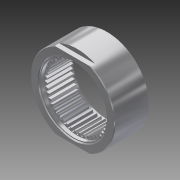
# Autodesk Inventor part: P60 Ring Gear 1-Stage
Saved by Autodesk Inventor 2014 SP1 (Build 180222100, 222)
## iProperties
Created: 2012-01-14
Part Number: P60 Ring Gear 1-Stage
Material: Aluminum 6061
Document SubType Name: Modeling
Designer: Moses
Density: 2.71 g/cm^3
Mass: 18.5911 g
Surface Area: 48.1148 cm^2
Volume: 6.86017 cm^3
Appearance: Aluminum - Polished
Author: Moses
Autodesk Inventor part; units mm, degrees
ref_plane "YZ Plane" through (0, 0, 0) normal (1, 0, 0) x (0, 1, 0)
ref_plane "XZ Plane" through (0, 0, 0) normal (0, 1, 0) x (-1, 0, 0)
sketch "Sketch1" plane through (0, 0, 0) normal (0, 0, 1) x (1, 0, 0)
  circle A0 centre (0, 0) radius 18.415
  circle A1 centre (0, 0) radius 14.9225
  dimension "d0" = 36.83
  dimension "d1" = 29.845
  constraints: 2 centre point, 2 coincident
  measures "d0" diameter of A0
  measures "d1" diameter of A1
extrude "Extrusion1" add sketch "Sketch1" along normal blind 15.24
chamfer "Chamfer1" distance 0.254 angle 45 4 edges at (-18.415, 0, 15.24) (-14.9225, 0, 15.24) (-18.415, 0, 0) (-14.9225, 0, 0)
sketch "Sketch2" plane through (0, 0, 15.24) normal (0, 0, 1) x (1, 0, 0)
  circle A0 centre (0, 0) radius 18.415 projected
  line L0 (-7.9375, 16.6165) -> (7.9375, 16.6165)
  line L1 (-7.9375, -16.6165) -> (7.9375, -16.6165)
  dimension "d7" = 15.875
  dimension "d16" = 36.83
  constraints: 4 end point, 4 point on circle, 2 parallel, 1 horizontal
  measures "d7" distance of L1.start L1.end
  measures "d16" diameter of A0
extrude "Extrusion2" cut sketch "Sketch2" against normal blind 2 contours L0 A0 | A0 L1
ref_plane "Work Plane1" through (0, 0, 7.62) normal (0, 0, 1) x (1, 0, 0)
sketch "Sketch3" plane through (0, 0, 7.62) normal (0, 0, 1) x (1, 0, 0)
  arc A0 (2.2292, -14.0746) -> (2.4908, -12.8141) centre (-3.3575, -12.2576) ccw
  arc A1 (1.7366, -14.1438) -> (2.2292, -14.0746) centre (0, 0) ccw
  arc A2 (1.1377, -13.0043) -> (1.7366, -14.1438) centre (6.6061, -10.8573) ccw
  arc A3 (0.6832, -13.0361) -> (1.1377, -13.0043) centre (0, 0) ccw
  arc A4 (0.2487, -14.2478) -> (0.6832, -13.0361) centre (-5.0308, -11.671) ccw
  arc A5 (-0.2487, -14.2478) -> (0.2487, -14.2478) centre (0, 0) ccw
  arc A6 (-0.6832, -13.0361) -> (-0.2487, -14.2478) centre (5.0308, -11.671) ccw
  arc A7 (-1.1377, -13.0043) -> (-0.6832, -13.0361) centre (0, 0) ccw
  arc A8 (-1.7366, -14.1438) -> (-1.1377, -13.0043) centre (-6.6061, -10.8573) ccw
  arc A9 (-2.2292, -14.0746) -> (-1.7366, -14.1438) centre (0, 0) ccw
  arc A10 (-2.4908, -12.8141) -> (-2.2292, -14.0746) centre (3.3575, -12.2576) ccw
  arc A11 (-2.9365, -12.7194) -> (-2.4908, -12.8141) centre (0, 0) ccw
  arc A12 (-3.6882, -13.7644) -> (-2.9365, -12.7194) centre (-8.0529, -9.8322) ccw
  arc A13 (-4.1663, -13.6273) -> (-3.6882, -13.7644) centre (0, 0) ccw
  arc A14 (-4.25, -12.3428) -> (-4.1663, -13.6273) centre (1.6189, -12.6056) ccw
  arc A15 (-4.6781, -12.1869) -> (-4.25, -12.3428) centre (0, 0) ccw
  arc A16 (-5.5679, -13.1172) -> (-4.6781, -12.1869) centre (-9.3429, -8.6158) ccw
  arc A17 (-6.0223, -12.9149) -> (-5.5679, -13.1172) centre (0, 0) ccw
  arc A18 (-5.9264, -11.6312) -> (-6.0223, -12.9149) centre (-0.1512, -12.7082) ccw
  arc A19 (-6.3287, -11.4173) -> (-5.9264, -11.6312) centre (0, 0) ccw
  arc A20 (-7.3393, -12.2146) -> (-6.3287, -11.4173) centre (-10.451, -7.2317) ccw
  arc A21 (-7.7611, -11.9511) -> (-7.3393, -12.2146) centre (0, 0) ccw
  arc A22 (-7.4874, -10.6932) -> (-7.7611, -11.9511) centre (-1.9183, -12.5635) ccw
  arc A23 (-7.8561, -10.4254) -> (-7.4874, -10.6932) centre (0, 0) ccw
  arc A24 (-8.9678, -11.0743) -> (-7.8561, -10.4254) centre (-11.3558, -5.7068) ccw
  arc A25 (-9.3488, -10.7546) -> (-8.9678, -11.0743) centre (0, 0) ccw
  arc A26 (-8.9028, -9.5471) -> (-9.3488, -10.7546) centre (-3.6482, -12.1742) ccw
  arc A27 (-9.2305, -9.2305) -> (-8.9028, -9.5471) centre (0, 0) ccw
  arc A28 (-10.4218, -9.7185) -> (-9.2305, -9.2305) centre (-12.0395, -4.0708) ccw
  arc A29 (-10.7546, -9.3488) -> (-10.4218, -9.7185) centre (0, 0) ccw
  arc A30 (-10.1448, -8.2151) -> (-10.7546, -9.3488) centre (-5.307, -11.548) ccw
  arc A31 (-10.4254, -7.8561) -> (-10.1448, -8.2151) centre (0, 0) ccw
  arc A32 (-11.6729, -8.1735) -> (-10.4254, -7.8561) centre (-12.4889, -2.3556) ccw
  arc A33 (-11.9511, -7.7611) -> (-11.6729, -8.1735) centre (0, 0) ccw
  arc A34 (-11.1894, -6.7233) -> (-11.9511, -7.7611) centre (-6.8625, -10.6971) ccw
  arc A35 (-11.4173, -6.3287) -> (-11.1894, -6.7233) centre (0, 0) ccw
  arc A36 (-12.6968, -6.4694) -> (-11.4173, -6.3287) centre (-12.6952, -0.5946) ccw
  arc A37 (-12.9149, -6.0223) -> (-12.6968, -6.4694) centre (0, 0) ccw
  arc A38 (-12.0162, -5.1006) -> (-12.9149, -6.0223) centre (-8.2845, -9.6379) ccw
  arc A39 (-12.1869, -4.6781) -> (-12.0162, -5.1006) centre (0, 0) ccw
  arc A40 (-13.4736, -4.6393) -> (-12.1869, -4.6781) centre (-12.6544, 1.178) ccw
  arc A41 (-13.6273, -4.1663) -> (-13.4736, -4.6393) centre (0, 0) ccw
  arc A42 (-12.6092, -3.3786) -> (-13.6273, -4.1663) centre (-9.5452, -8.3911) ccw
  arc A43 (-12.7194, -2.9365) -> (-12.6092, -3.3786) centre (0, 0) ccw
  arc A44 (-13.9882, -2.719) -> (-12.7194, -2.9365) centre (-12.3673, 2.9277) ccw
  arc A45 (-14.0746, -2.2292) -> (-13.9882, -2.719) centre (0, 0) ccw
  arc A46 (-12.9567, -1.5909) -> (-14.0746, -2.2292) centre (-10.6201, -6.981) ccw
  arc A47 (-13.0043, -1.1377) -> (-12.9567, -1.5909) centre (0, 0) ccw
  arc A48 (-14.2305, -0.7458) -> (-13.0043, -1.1377) centre (-11.8395, 4.6204) ccw
  arc A49 (-14.2478, -0.2487) -> (-14.2305, -0.7458) centre (0, 0) ccw
  arc A50 (-13.052, 0.2278) -> (-14.2478, -0.2487) centre (-11.4883, -5.435) ccw
  arc A51 (-13.0361, 0.6832) -> (-13.052, 0.2278) centre (0, 0) ccw
  arc A52 (-14.1958, 1.242) -> (-13.0361, 0.6832) centre (-11.0812, 6.2232) ccw
  arc A53 (-14.1438, 1.7366) -> (-14.1958, 1.242) centre (0, 0) ccw
  arc A54 (-12.8932, 2.0421) -> (-14.1438, 1.7366) centre (-12.1329, -3.7833) ccw
  arc A55 (-12.8141, 2.4908) -> (-12.8932, 2.0421) centre (0, 0) ccw
  arc A56 (-13.8848, 3.2056) -> (-12.8141, 2.4908) centre (-10.1073, 7.7048) ccw
  arc A57 (-13.7644, 3.6882) -> (-13.8848, 3.2056) centre (0, 0) ccw
  arc A58 (-12.4836, 3.8166) -> (-13.7644, 3.6882) centre (-12.5414, -2.0579) ccw
  arc A59 (-12.3428, 4.25) -> (-12.4836, 3.8166) centre (0, 0) ccw
  arc A60 (-13.3035, 5.1067) -> (-12.3428, 4.25) centre (-8.9366, 9.0365) ccw
  arc A61 (-13.1172, 5.5679) -> (-13.3035, 5.1067) centre (0, 0) ccw
  arc A62 (-11.8309, 5.5168) -> (-13.1172, 5.5679) centre (-12.7057, -0.2924) ccw
  arc A63 (-11.6312, 5.9264) -> (-11.8309, 5.5168) centre (0, 0) ccw
  arc A64 (-12.4633, 6.9085) -> (-11.6312, 5.9264) centre (-7.592, 10.1923) ccw
  arc A65 (-12.2146, 7.3393) -> (-12.4633, 6.9085) centre (0, 0) ccw
  arc A66 (-10.948, 7.1097) -> (-12.2146, 7.3393) centre (-12.6228, 1.4787) ccw
  arc A67 (-10.6932, 7.4874) -> (-10.948, 7.1097) centre (0, 0) ccw
  arc A68 (-11.3806, 8.5759) -> (-10.6932, 7.4874) centre (-6.0996, 11.1497) ccw
  arc A69 (-11.0743, 8.9678) -> (-11.3806, 8.5759) centre (0, 0) ccw
  arc A70 (-9.852, 8.5642) -> (-11.0743, 8.9678) centre (-12.2941, 3.2211) ccw
  arc A71 (-9.5471, 8.9028) -> (-9.852, 8.5642) centre (0, 0) ccw
  arc A72 (-10.0763, 10.0763) -> (-9.5471, 8.9028) centre (-4.4885, 11.8901) ccw
  arc A73 (-9.7185, 10.4218) -> (-10.0763, 10.0763) centre (0, 0) ccw
  arc A74 (-8.5642, 9.852) -> (-9.7185, 10.4218) centre (-11.7262, 4.9007) ccw
  arc A75 (-8.2151, 10.1448) -> (-8.5642, 9.852) centre (0, 0) ccw
  arc A76 (-8.5759, 11.3806) -> (-8.2151, 10.1448) centre (-2.79, 12.3991) ccw
  arc A77 (-8.1735, 11.6729) -> (-8.5759, 11.3806) centre (0, 0) ccw
  arc A78 (-7.1097, 10.948) -> (-8.1735, 11.6729) centre (-10.93, 6.485) ccw
  arc A79 (-6.7233, 11.1894) -> (-7.1097, 10.948) centre (0, 0) ccw
  arc A80 (-6.9085, 12.4633) -> (-6.7233, 11.1894) centre (-1.0373, 12.6667) ccw
  arc A81 (-6.4694, 12.6968) -> (-6.9085, 12.4633) centre (0, 0) ccw
  arc A82 (-5.5168, 11.8309) -> (-6.4694, 12.6968) centre (-9.9211, 7.9431) ccw
  arc A83 (-5.1006, 12.0162) -> (-5.5168, 11.8309) centre (0, 0) ccw
  arc A84 (-5.1067, 13.3035) -> (-5.1006, 12.0162) centre (0.7357, 12.6878) ccw
  arc A85 (-4.6393, 13.4736) -> (-5.1067, 13.3035) centre (0, 0) ccw
  arc A86 (-3.8166, 12.4836) -> (-4.6393, 13.4736) centre (-8.7191, 9.2465) ccw
  arc A87 (-3.3786, 12.6092) -> (-3.8166, 12.4836) centre (0, 0) ccw
  arc A88 (-3.2056, 13.8848) -> (-3.3786, 12.6092) centre (2.4943, 12.4619) ccw
  arc A89 (-2.719, 13.9882) -> (-3.2056, 13.8848) centre (0, 0) ccw
  arc A90 (-2.0421, 12.8932) -> (-2.719, 13.9882) centre (-7.3474, 10.37) ccw
  arc A91 (-1.5909, 12.9567) -> (-2.0421, 12.8932) centre (0, 0) ccw
  arc A92 (-1.242, 14.1958) -> (-1.5909, 12.9567) centre (4.2044, 11.9935) ccw
  arc A93 (-0.7458, 14.2305) -> (-1.242, 14.1958) centre (0, 0) ccw
  arc A94 (-0.2278, 13.052) -> (-0.7458, 14.2305) centre (-5.8327, 11.2916) ccw
  arc A95 (0.2278, 13.052) -> (-0.2278, 13.052) centre (0, 0) ccw
  arc A96 (0.7458, 14.2305) -> (0.2278, 13.052) centre (5.8327, 11.2916) ccw
  arc A97 (1.242, 14.1958) -> (0.7458, 14.2305) centre (0, 0) ccw
  arc A98 (1.5909, 12.9567) -> (1.242, 14.1958) centre (-4.2044, 11.9935) ccw
  arc A99 (2.0421, 12.8932) -> (1.5909, 12.9567) centre (0, 0) ccw
  arc A100 (2.719, 13.9882) -> (2.0421, 12.8932) centre (7.3474, 10.37) ccw
  arc A101 (3.2056, 13.8848) -> (2.719, 13.9882) centre (0, 0) ccw
  arc A102 (3.3786, 12.6092) -> (3.2056, 13.8848) centre (-2.4943, 12.4619) ccw
  arc A103 (3.8166, 12.4836) -> (3.3786, 12.6092) centre (0, 0) ccw
  arc A104 (4.6393, 13.4736) -> (3.8166, 12.4836) centre (8.7191, 9.2465) ccw
  arc A105 (5.1067, 13.3035) -> (4.6393, 13.4736) centre (0, 0) ccw
  arc A106 (5.1006, 12.0162) -> (5.1067, 13.3035) centre (-0.7357, 12.6878) ccw
  arc A107 (5.5168, 11.8309) -> (5.1006, 12.0162) centre (0, 0) ccw
  arc A108 (6.4694, 12.6968) -> (5.5168, 11.8309) centre (9.9211, 7.9431) ccw
  arc A109 (6.9085, 12.4633) -> (6.4694, 12.6968) centre (0, 0) ccw
  arc A110 (6.7233, 11.1894) -> (6.9085, 12.4633) centre (1.0373, 12.6667) ccw
  arc A111 (7.1097, 10.948) -> (6.7233, 11.1894) centre (0, 0) ccw
  arc A112 (8.1735, 11.6729) -> (7.1097, 10.948) centre (10.93, 6.485) ccw
  arc A113 (8.5759, 11.3806) -> (8.1735, 11.6729) centre (0, 0) ccw
  arc A114 (8.2151, 10.1448) -> (8.5759, 11.3806) centre (2.79, 12.3991) ccw
  arc A115 (8.5642, 9.852) -> (8.2151, 10.1448) centre (0, 0) ccw
  arc A116 (9.7185, 10.4218) -> (8.5642, 9.852) centre (11.7262, 4.9007) ccw
  arc A117 (10.0763, 10.0763) -> (9.7185, 10.4218) centre (0, 0) ccw
  arc A118 (9.5471, 8.9028) -> (10.0763, 10.0763) centre (4.4885, 11.8901) ccw
  arc A119 (9.852, 8.5642) -> (9.5471, 8.9028) centre (0, 0) ccw
  arc A120 (11.0743, 8.9678) -> (9.852, 8.5642) centre (12.2941, 3.2211) ccw
  arc A121 (11.3806, 8.5759) -> (11.0743, 8.9678) centre (0, 0) ccw
  arc A122 (10.6932, 7.4874) -> (11.3806, 8.5759) centre (6.0996, 11.1497) ccw
  arc A123 (10.948, 7.1097) -> (10.6932, 7.4874) centre (0, 0) ccw
  arc A124 (12.2146, 7.3393) -> (10.948, 7.1097) centre (12.6228, 1.4787) ccw
  arc A125 (12.4633, 6.9085) -> (12.2146, 7.3393) centre (0, 0) ccw
  arc A126 (11.6312, 5.9264) -> (12.4633, 6.9085) centre (7.592, 10.1923) ccw
  arc A127 (11.8309, 5.5168) -> (11.6312, 5.9264) centre (0, 0) ccw
  arc A128 (13.1172, 5.5679) -> (11.8309, 5.5168) centre (12.7057, -0.2924) ccw
  arc A129 (13.3035, 5.1067) -> (13.1172, 5.5679) centre (0, 0) ccw
  arc A130 (12.3428, 4.25) -> (13.3035, 5.1067) centre (8.9366, 9.0365) ccw
  arc A131 (12.4836, 3.8166) -> (12.3428, 4.25) centre (0, 0) ccw
  arc A132 (13.7644, 3.6882) -> (12.4836, 3.8166) centre (12.5414, -2.0579) ccw
  arc A133 (13.8848, 3.2056) -> (13.7644, 3.6882) centre (0, 0) ccw
  arc A134 (12.8141, 2.4908) -> (13.8848, 3.2056) centre (10.1073, 7.7048) ccw
  arc A135 (12.8932, 2.0421) -> (12.8141, 2.4908) centre (0, 0) ccw
  arc A136 (14.1438, 1.7366) -> (12.8932, 2.0421) centre (12.1329, -3.7833) ccw
  arc A137 (14.1958, 1.242) -> (14.1438, 1.7366) centre (0, 0) ccw
  arc A138 (13.0361, 0.6832) -> (14.1958, 1.242) centre (11.0812, 6.2232) ccw
  arc A139 (13.052, 0.2278) -> (13.0361, 0.6832) centre (0, 0) ccw
  arc A140 (14.2478, -0.2487) -> (13.052, 0.2278) centre (11.4883, -5.435) ccw
  arc A141 (14.2305, -0.7458) -> (14.2478, -0.2487) centre (0, 0) ccw
  arc A142 (13.0043, -1.1377) -> (14.2305, -0.7458) centre (11.8395, 4.6204) ccw
  arc A143 (12.9567, -1.5909) -> (13.0043, -1.1377) centre (0, 0) ccw
  arc A144 (14.0746, -2.2292) -> (12.9567, -1.5909) centre (10.6201, -6.981) ccw
  arc A145 (13.9882, -2.719) -> (14.0746, -2.2292) centre (0, 0) ccw
  arc A146 (12.7194, -2.9365) -> (13.9882, -2.719) centre (12.3673, 2.9277) ccw
  arc A147 (12.6092, -3.3786) -> (12.7194, -2.9365) centre (0, 0) ccw
  arc A148 (13.6273, -4.1663) -> (12.6092, -3.3786) centre (9.5452, -8.3911) ccw
  arc A149 (13.4736, -4.6393) -> (13.6273, -4.1663) centre (0, 0) ccw
  arc A150 (12.1869, -4.6781) -> (13.4736, -4.6393) centre (12.6544, 1.178) ccw
  arc A151 (12.0162, -5.1006) -> (12.1869, -4.6781) centre (0, 0) ccw
  arc A152 (12.9149, -6.0223) -> (12.0162, -5.1006) centre (8.2845, -9.6379) ccw
  arc A153 (12.6968, -6.4694) -> (12.9149, -6.0223) centre (0, 0) ccw
  arc A154 (11.4173, -6.3287) -> (12.6968, -6.4694) centre (12.6952, -0.5946) ccw
  arc A155 (11.1894, -6.7233) -> (11.4173, -6.3287) centre (0, 0) ccw
  arc A156 (11.9511, -7.7611) -> (11.1894, -6.7233) centre (6.8625, -10.6971) ccw
  arc A157 (11.6729, -8.1735) -> (11.9511, -7.7611) centre (0, 0) ccw
  arc A158 (10.4254, -7.8561) -> (11.6729, -8.1735) centre (12.4889, -2.3556) ccw
  arc A159 (10.1448, -8.2151) -> (10.4254, -7.8561) centre (0, 0) ccw
  arc A160 (10.7546, -9.3488) -> (10.1448, -8.2151) centre (5.307, -11.548) ccw
  arc A161 (10.4218, -9.7185) -> (10.7546, -9.3488) centre (0, 0) ccw
  arc A162 (9.2305, -9.2305) -> (10.4218, -9.7185) centre (12.0395, -4.0708) ccw
  arc A163 (8.9028, -9.5471) -> (9.2305, -9.2305) centre (0, 0) ccw
  arc A164 (9.3488, -10.7546) -> (8.9028, -9.5471) centre (3.6482, -12.1742) ccw
  arc A165 (8.9678, -11.0743) -> (9.3488, -10.7546) centre (0, 0) ccw
  arc A166 (7.8561, -10.4254) -> (8.9678, -11.0743) centre (11.3558, -5.7068) ccw
  arc A167 (7.4874, -10.6932) -> (7.8561, -10.4254) centre (0, 0) ccw
  arc A168 (7.7611, -11.9511) -> (7.4874, -10.6932) centre (1.9183, -12.5635) ccw
  arc A169 (7.3393, -12.2146) -> (7.7611, -11.9511) centre (0, 0) ccw
  arc A170 (6.3287, -11.4173) -> (7.3393, -12.2146) centre (10.451, -7.2317) ccw
  arc A171 (5.9264, -11.6312) -> (6.3287, -11.4173) centre (0, 0) ccw
  arc A172 (6.0223, -12.9149) -> (5.9264, -11.6312) centre (0.1512, -12.7082) ccw
  arc A173 (5.5679, -13.1172) -> (6.0223, -12.9149) centre (0, 0) ccw
  arc A174 (4.6781, -12.1869) -> (5.5679, -13.1172) centre (9.3429, -8.6158) ccw
  arc A175 (4.25, -12.3428) -> (4.6781, -12.1869) centre (0, 0) ccw
  arc A176 (4.1663, -13.6273) -> (4.25, -12.3428) centre (-1.6189, -12.6056) ccw
  arc A177 (3.6882, -13.7644) -> (4.1663, -13.6273) centre (0, 0) ccw
  arc A178 (2.9365, -12.7194) -> (3.6882, -13.7644) centre (8.0529, -9.8322) ccw
  arc A179 (2.4908, -12.8141) -> (2.9365, -12.7194) centre (0, 0) ccw
  circle A180 centre (0, 0) radius 14.9225 projected
  circle A181 centre (0, 0) radius 14.478
  dimension "d10" = 28.956
  constraints: 360 point on circle, 181 centre point, 1 coincident, 542 other
  measures "d10" diameter of A181
extrude "Extrusion3" add sketch "Sketch3" along normal mid plane 14.24 contours A180
extrude "Extrusion4" add sketch "Sketch3" along normal mid plane 11.24 contours A181
body "Solid1"
